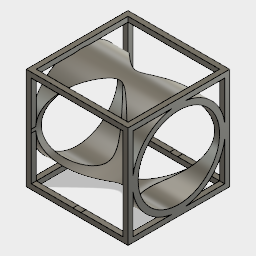
cube v3 (Autodesk Fusion 360 design; units mm, degrees)
Autodesk Fusion 360 part; units mm, degrees
sketch "Sketch1" plane through (0, 0, 0) normal (0, 1, 0) x (1, 0, 0)
  line L0 (-35, 18) -> (-29, 18)
  line L1 (-29, 18) -> (-29, 12)
  line L2 (-29, 12) -> (-35, 12)
  line L3 (-35, 12) -> (-35, 18)
sketch "Sketch2" plane through (0, 5, 0) normal (0, 1, 0) x (-1, 0, 0)
  line L0 (35, -12) -> (29, -12)
  line L1 (29, -12) -> (29, -18)
  line L2 (29, -18) -> (35, -18)
  line L3 (35, -18) -> (35, -12)
  line L4 (30, 0) -> (40, 0)
  line L5 (40, 0) -> (40, -10)
  line L6 (40, -10) -> (30, -10)
  line L7 (30, -10) -> (30, 0)
extrude "Extrude2" add sketch "Sketch2" along normal blind 10 contours L4 L5 L6 L7 makes body 1
sketch "Sketch3" plane through (0, 15, 0) normal (0, 1, 0) x (-1, 0, 0)
  line L0 (30, -10) -> (40, -10)
  line L1 (40, -10) -> (40, 0)
  line L2 (40, 0) -> (30, 0)
  line L3 (30, 0) -> (30, -10)
  line L4 (39.5, -9.5) -> (30.5, -9.5)
  line L5 (30.5, -9.5) -> (30.5, -0.5)
  line L6 (30.5, -0.5) -> (39.5, -0.5)
  line L7 (39.5, -0.5) -> (39.5, -9.5)
extrude "Extrude3" cut sketch "Sketch3" against normal blind 18 contours L4 L5 L6 L7 bodies 1
sketch "Sketch4" plane through (-30, 0, 0) normal (1, 0, 0) x (0, 0, -1)
  line L0 (0, 5) -> (10, 5)
  line L1 (10, 5) -> (10, 15)
  line L2 (10, 15) -> (0, 15)
  line L3 (0, 15) -> (0, 5)
  line L4 (0.5, 14.5) -> (9.5, 14.5)
  line L5 (9.5, 14.5) -> (9.5, 5.5)
  line L6 (9.5, 5.5) -> (0.5, 5.5)
  line L7 (0.5, 5.5) -> (0.5, 14.5)
  line L8 (0.5, 15) -> (0.5, 5)
  line L9 (9.5, 15) -> (9.5, 5)
extrude "Extrude4" cut sketch "Sketch4" against normal blind 16 contours L4 L5 L6 L7 L8 L9 bodies 1
sketch "Sketch5" plane through (0, 0, 0) normal (0, 0, 1) x (1, 0, 0)
  line L0 (-40, 5) -> (-30, 5)
  line L1 (-30, 5) -> (-30, 15)
  line L2 (-30, 15) -> (-40, 15)
  line L3 (-40, 15) -> (-40, 5)
  line L4 (-39.5, 14.5) -> (-30.5, 14.5)
  line L5 (-30.5, 14.5) -> (-30.5, 6)
  line L6 (-30.5, 6) -> (-39.5, 6)
  line L7 (-39.5, 6) -> (-39.5, 14.5)
  dimension "d9" = 8.5
  measures "d9" distance of L4.start L6.end
extrude "Extrude5" cut sketch "Sketch5" against normal blind 23 contours L4 L5 L6 L7 bodies 1
sketch "Sketch6" plane through (0, 0, -10) normal (0, 0, -1) x (-1, 0, 0)
  line L0 (30.5, 6) -> (30.5, 14.5)
  line L1 (30.5, 14.5) -> (39.5, 14.5)
  line L2 (39.5, 14.5) -> (39.5, 6)
  line L3 (39.5, 6) -> (30.5, 6)
  line L4 (30, 5) -> (40, 5)
  line L5 (40, 5) -> (40, 15)
  line L6 (40, 15) -> (30, 15)
  line L7 (30, 15) -> (30, 5)
  line L8 (30.5, 6) -> (39.5, 6)
  line L9 (39.5, 6) -> (39.5, 5.5)
  line L10 (39.5, 5.5) -> (30.5, 5.5)
  line L11 (30.5, 5.5) -> (30.5, 6)
  point P0 (39.5, 5.5)
extrude "Extrude6" cut sketch "Sketch6" against normal blind 26.5 contours L3 L8 L9 L10 L11 bodies 1
sketch "Sketch7" plane through (0, 0, 0) normal (1, 0, 0) x (0, 0, -1)
sketch "Sketch8" plane through (0, 0, 0) normal (1, 0, 0) x (0, 0, -1)
  circle A0 centre (5, 10) radius 4.5568
  dimension "d15" = 9.1136
  measures "d15" diameter of A0
extrude "Extrude7" add sketch "Sketch8" along normal blind 10 separate body makes body 2
move_body "Move1" bodies 2 to x (1, 0, 0) y (0, 1, 0) z (0, 0, 1) at (-40, 0, 2)
move_body "Move2" bodies 2 to x (1, 0, 0) y (0, 1, 0) z (0, 0, 1) at (0, 0, -2)
sketch "Sketch9" plane through (-30, 0, 0) normal (1, 0, 0) x (0, 0, -1)
  circle A0 centre (5, 10) radius 4.5568
  circle A1 centre (5, 10) radius 4
  dimension "d24" = 8
  measures "d24" diameter of A1
extrude "Extrude8" cut sketch "Sketch9" against normal blind 18 contours A1 bodies 2
sketch "Sketch10" plane through (0, 0, 0) normal (0, 0, 1) x (1, 0, 0)
  circle A0 centre (-35.0032, 9.983) radius 4.5
  dimension "d27" = 9
  measures "d27" diameter of A0
extrude "Extrude9" cut sketch "Sketch10" against normal blind 22 bodies 1 2
combine "Combine1" operation add target body 1 tool bodies 2
